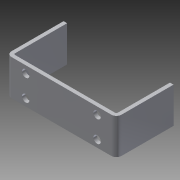
# Autodesk Inventor part: M - Upper Rail Connector Bracket 1
Saved by Autodesk Inventor 2013 (Build 170138000, 138)
## iProperties
Created: 2013-02-17
Part Number: M - Upper Rail Connector Bracket 1
Material: Aluminum 6061
Document SubType Name: Sheet Metal
Designer: Moses
Density: 2.71 g/cm^3
Mass: 50.8866 g
Surface Area: 135.036 cm^2
Volume: 18.7774 cm^3
Sheet Metal Rule: Default
Author: Moses
Autodesk Inventor part; units mm, degrees
ref_plane "YZ Plane" through (0, 0, 0) normal (1, 0, 0) x (0, 1, 0)
ref_plane "XZ Plane" through (0, 0, 0) normal (0, 1, 0) x (-1, 0, 0)
ref_plane "XY Plane" through (0, 0, 0) normal (0, 0, 1) x (1, 0, 0)
sketch "Sketch1" plane through (0, 0, 0) normal (0, 0, 1) x (1, 0, 0)
  line L0 (0, 0) -> (88.9, 0)
  line L1 (88.9, 0) -> (88.9, 31.75)
  line L2 (88.9, 31.75) -> (0, 31.75)
  line L3 (0, 31.75) -> (0, 0)
  circle A0 centre (12.7, 25.4) radius 3.302
  circle A1 centre (76.2, 25.4) radius 3.302
  circle A2 centre (12.7, 6.35) radius 3.302
  circle A3 centre (76.2, 6.35) radius 3.302
  line L4 (12.7, 25.4) -> (76.2, 25.4) construction
  line L5 (44.45, 31.75) -> (44.45, 0) construction
  point P0 (44.45, 25.4)
  dimension "d0" = 88.9
  dimension "d2" = 31.75
  dimension "d5" = 63.5
  dimension "d8" = 19.05
  dimension "d11" = 6.35
  dimension "d12" = 6.604
  measures "d0" distance of L1.end L2.end
  measures "d2" distance of L2.end L0.start
  measures "d5" distance of L4.start L4.end
  measures "d8" distance of L4.start A2.centre
  measures "d11" distance from line of L2 L4.start
  measures "d12" diameter of A0
extrude "Plate1" add sketch "Sketch1" along normal blind 3.175
sketch "Sketch2" plane through (90.17, 0, -1.27) normal (1, 0, 0) x (0, 1, 0)
  line L0 (31.75, 0) -> (0, 0)
  line L1 (0, 0) -> (0, -46.355)
  line L2 (0, -46.355) -> (31.75, -46.355)
  line L3 (31.75, -46.355) -> (31.75, 0)
  constraints: 6 end point, 1 horizontal, 1 perpendicular, 1 vertical
edge flange "Flange1" height 50.8 angle 90 thickness 3.175 bend radius 1.27 thickness toward (1, 0, 0) relief straight relief width 3.175 relief depth 1.5875 corner gap 3.175 corner form 0 edges at (88.9, 15.875, 0) (0, 15.875, 0) wall of the first edge with corners at (90.17, 31.75, -1.27) (90.17, 0, -1.27) (90.17, 0, -47.625) (90.17, 31.75, -47.625)
bend "Bend1"
corner "Corner1"
equation "\"d16\" = BendReliefWidth"
equation "\"d17\" = BendReliefDepth"
equation "\"d18\" = MinimumRemnant"
equation "\"d19\" = BendRadius"
equation "\"d23\" = CornerReliefSize"
equation "\"d24\" = GapSize"
equation "\"d25\" = JacobiRadiusSize"
equation "\"BendRadius\" = Thickness"
equation "\"BendReliefWidth\" = Thickness"
equation "\"BendReliefDepth\" = 0.5 * Thickness"
equation "\"CornerReliefSize\" = 4 * Thickness"
equation "\"MinimumRemnant\" = 2 * Thickness"
equation "\"TransitionRadius\" = BendRadius"
equation "\"JacobiRadiusSize\" = Thickness"
equation "\"GapSize\" = Thickness"
equation "\"d15\" = BendRadius"
equation "\"Thickness\" = 3.175"
body "Solid2"
